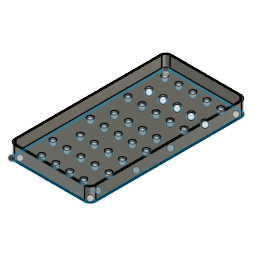
Trey (Autodesk Fusion 360 design; units mm, degrees)
part number: 2026-07-11-13-08-03-069
Autodesk Fusion 360 part; units mm, degrees
sketch "Sketch1" plane through (0, 0, 0) normal (0, 0, 1) x (1, 0, 0)
  line L0 (-175, 70) -> (75, 70)
  line L1 (90, 85) -> (90, 605)
  line L2 (75, 620) -> (-175, 620)
  line L3 (-190, 605) -> (-190, 85)
  arc A0 (90, 605) -> (75, 620) centre (75, 605) ccw
  arc A1 (-175, 620) -> (-190, 605) centre (-175, 605) ccw
  arc A2 (-190, 85) -> (-175, 70) centre (-175, 85) ccw
  arc A3 (75, 70) -> (90, 85) centre (75, 85) ccw
  line L4 (-195, 605) -> (-195, 85)
  arc A4 (-195, 85) -> (-175, 65) centre (-175, 85) ccw
  line L5 (-175, 65) -> (75, 65)
  arc A5 (75, 65) -> (95, 85) centre (75, 85) ccw
  line L6 (95, 85) -> (95, 605)
  arc A6 (95, 605) -> (75, 625) centre (75, 605) ccw
  line L7 (75, 625) -> (-175, 625)
  arc A7 (-175, 625) -> (-195, 605) centre (-175, 605) ccw
  circle A8 centre (-160.8581, 587.3244) radius 10
  circle A9 centre (-110.8581, 587.3244) radius 10
  circle A10 centre (-60.8581, 587.3244) radius 10
  circle A11 centre (-10.8581, 587.3244) radius 10
  circle A12 centre (39.1419, 587.3244) radius 10
  circle A13 centre (-148.0256, 518.1715) radius 10
  circle A14 centre (-98.0256, 518.1715) radius 10
  circle A15 centre (-48.0256, 518.1715) radius 10
  circle A16 centre (1.9744, 518.1715) radius 10
  circle A17 centre (51.9744, 518.1715) radius 10
  circle A18 centre (-148.0256, 518.1715) radius 10
  circle A19 centre (-98.0256, 518.1715) radius 10
  circle A20 centre (-48.0256, 518.1715) radius 10
  circle A21 centre (1.9744, 518.1715) radius 10
  circle A22 centre (-148.0256, 518.1715) radius 10
  circle A23 centre (-98.0256, 518.1715) radius 10
  circle A24 centre (-48.0256, 518.1715) radius 10
  circle A25 centre (1.9744, 518.1715) radius 10
  circle A26 centre (51.9744, 518.1715) radius 10
  circle A27 centre (-163.7098, 458.9995) radius 10
  circle A28 centre (-113.7098, 458.9995) radius 10
  circle A29 centre (-63.7098, 458.9995) radius 10
  circle A30 centre (-13.7098, 458.9995) radius 10
  circle A31 centre (36.2902, 458.9995) radius 10
  circle A32 centre (-136.6189, 383.4303) radius 10
  circle A33 centre (-86.6189, 383.4303) radius 10
  circle A34 centre (-36.6189, 383.4303) radius 10
  circle A35 centre (13.3811, 383.4303) radius 10
  circle A36 centre (63.3811, 383.4303) radius 10
  circle A37 centre (-164.4775, 324.9712) radius 10
  circle A38 centre (-114.4775, 324.9712) radius 10
  circle A39 centre (-64.4775, 324.9712) radius 10
  circle A40 centre (-14.4775, 324.9712) radius 10
  circle A41 centre (35.5225, 324.9712) radius 10
  circle A42 centre (-129.4898, 254.3925) radius 10
  circle A43 centre (-79.4898, 254.3925) radius 10
  circle A44 centre (-29.4898, 254.3925) radius 10
  circle A45 centre (20.5102, 254.3925) radius 10
  circle A46 centre (70.5102, 254.3925) radius 10
  circle A47 centre (-162.2839, 189.5171) radius 10
  circle A48 centre (-112.2839, 189.5171) radius 10
  circle A49 centre (-62.2839, 189.5171) radius 10
  circle A50 centre (-12.2839, 189.5171) radius 10
  circle A51 centre (37.7161, 189.5171) radius 10
  circle A52 centre (-135.906, 123.2159) radius 10
  circle A53 centre (-85.906, 123.2159) radius 10
  circle A54 centre (-35.906, 123.2159) radius 10
  circle A55 centre (14.094, 123.2159) radius 10
  circle A56 centre (64.094, 123.2159) radius 10
  point P0 (-190, 70)
  point P1 (-190, 620)
  point P2 (51.9744, 518.1715)
  point P3 (51.9744, 518.1715)
  point P4 (-148.0256, 518.1715)
  point P5 (1.9744, 518.1715)
  point P6 (-98.0256, 518.1715)
  point P7 (-48.0256, 518.1715)
  dimension "d1" = 550
  dimension "d2" = 280
  dimension "d3" = 15
  dimension "d4" = 5
  dimension "d5" = 20
  dimension "d6" = 20
  dimension "d7" = 20
  dimension "d8" = 20
  dimension "d9" = 20
  dimension "d10" = 20
  dimension "d11" = 20
  dimension "d12" = 20
  dimension "d13" = 20
  dimension "d14" = 20
  dimension "d15" = 20
  dimension "d16" = 20
  dimension "d17" = 20
  dimension "d18" = 20
  dimension "d19" = 20
  dimension "d20" = 20
  dimension "d21" = 20
  dimension "d22" = 20
  dimension "d23" = 20
  dimension "d24" = 20
  dimension "d25" = 20
  dimension "d26" = 20
  dimension "d27" = 20
  dimension "d28" = 20
  dimension "d29" = 20
  dimension "d30" = 20
  dimension "d31" = 20
  dimension "d32" = 20
  dimension "d33" = 20
  dimension "d34" = 20
  dimension "d35" = 20
  dimension "d36" = 20
  dimension "d37" = 20
  dimension "d38" = 20
  dimension "d39" = 20
  dimension "d40" = 20
  dimension "d41" = 20
  dimension "d42" = 20
  dimension "d43" = 20
  dimension "d44" = 20
  dimension "d45" = 20
  dimension "d46" = 20
  dimension "d47" = 20
  dimension "d48" = 20
  dimension "d49" = 20
  dimension "d50" = 20
  dimension "d51" = 20
  dimension "d52" = 20
  dimension "d53" = 20
  constraint horizontal L0
  constraint vertical L1
  constraint horizontal L2
  constraint vertical L3
  constraint tangent L1 A0
  constraint tangent L2 A0
  constraint coincident P1 L2
  constraint coincident P1 L3
  constraint tangent L2 A1
  constraint tangent L3 A1
  constraint equal A0 A1
  constraint coincident P0 L0
  constraint coincident P0 L3
  constraint tangent L0 A2
  constraint tangent L3 A2
  constraint equal A0 A2
  constraint tangent L0 A3
  constraint tangent L1 A3
  constraint equal A0 A3
  measures "d1" distance of P0 P1
  measures "d2" distance of L1 L3
  measures "d3" radius of A0 A47.centre
  measures "d5" diameter of A8
  measures "d6" diameter of A9
  measures "d7" diameter of A10
  measures "d8" diameter of A11
  measures "d9" diameter of A12
  measures "d10" diameter of A13
  measures "d11" diameter of A14
  measures "d12" diameter of A15
  measures "d13" diameter of A16
  measures "d14" diameter of A17
  measures "d15" diameter of A18
  measures "d16" diameter of A19
  measures "d17" diameter of A20
  measures "d18" diameter of A21
  measures "d19" diameter of A22
  measures "d20" diameter of A23
  measures "d21" diameter of A24
  measures "d22" diameter of A25
  measures "d23" diameter of A26
  measures "d24" diameter of A29
  measures "d25" diameter of A27
  measures "d26" diameter of A30
  measures "d27" diameter of A28
  measures "d28" diameter of A31
  measures "d29" diameter of A34
  measures "d30" diameter of A32
  measures "d31" diameter of A35
  measures "d32" diameter of A33
  measures "d33" diameter of A36
  measures "d34" diameter of A39
  measures "d35" diameter of A37
  measures "d36" diameter of A40
  measures "d37" diameter of A38
  measures "d38" diameter of A41
  measures "d39" diameter of A44
  measures "d40" diameter of A42
  measures "d41" diameter of A45
  measures "d42" diameter of A43
  measures "d43" diameter of A46
  measures "d44" diameter of A49
  measures "d45" diameter of A47
  measures "d46" diameter of A50
  measures "d47" diameter of A48
  measures "d48" diameter of A51
  measures "d49" diameter of A54
  measures "d50" diameter of A52
  measures "d51" diameter of A55
  measures "d52" diameter of A53
  measures "d53" diameter of A56
extrude "Extrude1" add sketch "Sketch1" along normal blind 4 contours L4 A4 L5 A5 L6 A6 L7 A7 makes body 1
extrude "Extrude2" add sketch "Sketch1" along normal blind 50 separate body contours L4 A4 L5 A5 L6 A6 L7 A7 makes body 2
extrude "Extrude3" add sketch "Sketch1" along normal blind 10 contours L0 L1 L2 L3 A0 A1 A2 A3 bodies 1 2
extrude "Extrude4" add sketch "Sketch1" along normal blind 4 separate body contours L4 A4 L5 A5 L6 A6 L7 A7 makes body 3
